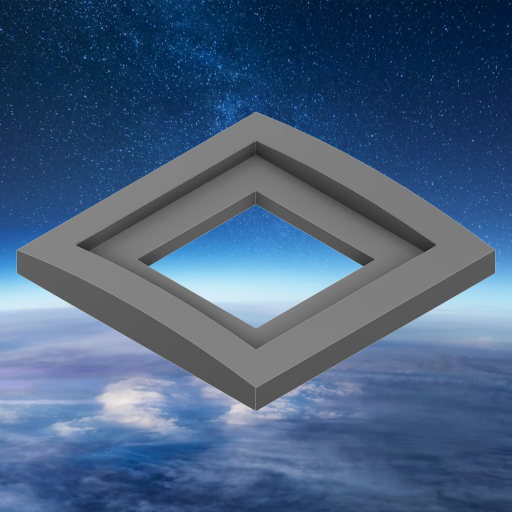
# Autodesk Inventor part: cooler_plate_socket
Saved by Autodesk Inventor 2023 (Build 270158000, 158)
## iProperties
Created: 2023-09-08
Part Number: cooler_plate_socket
Material: Acetal Resin, Black
Document SubType Name: Modeling
Designer: 310611102
Density: 1.425 g/cm^3
Appearance: Smooth - Black
Mass: 5.54751 g
Surface Area: 34.9135 cm^2
Volume: 3.89299 cm^3
Author: 310611102
Autodesk Inventor part; units mm, degrees
ref_plane "YZ Plane" through (0, 0, 0) normal (1, 0, 0) x (0, 1, 0)
ref_plane "XZ Plane" through (0, 0, 0) normal (0, 1, 0) x (-1, 0, 0)
ref_plane "XY Plane" through (0, 0, 0) normal (0, 0, 1) x (1, 0, 0)
sketch "Sketch1" plane through (0, 0, 0) normal (0, 0, 1) x (1, 0, 0)
  arc A0 (20, 123.3896) -> (-20, 123.3896) centre (0, 0) ccw
  line L0 (20, 120) -> (-20, 120)
  line L1 (-20, 120) -> (-20, 123.3896)
  line L2 (20, 120) -> (20, 123.3896)
  line L3 (0, 0) -> (0, 32.1156) construction
  point P0 (0, 125)
  dimension "d0" = 250
  dimension "d1" = 40
  dimension "d2" = 5
  constraints: 8 end point, 3 point on circle, 1 centre point, 1 coincident, 1 horizontal, 1 parallel, 1 perpendicular, 1 vertical, 1 other
  measures "d0" diameter of A0
  measures "d1" distance of L0.start L0.end
  measures "d2" distance from line of point (0, 125) L0
extrude "Extrusion1" add sketch "Sketch1" along normal blind 40
sketch "Sketch2" plane through (-20, 120, 0) normal (0, -1, 0) x (1, 0, 0)
  line L0 (4.85, 4.85) -> (35.15, 4.85)
  line L1 (35.15, 4.85) -> (35.15, 35.15)
  line L2 (35.15, 35.15) -> (4.85, 35.15)
  line L3 (4.85, 35.15) -> (4.85, 4.85)
  line L4 (4.85, 4.85) -> (35.15, 35.15) construction
  line L5 (35.15, 4.85) -> (4.85, 35.15) construction
  line L6 (40, 0) -> (40, 40) projected
  line L7 (40, 0) -> (0, 0) projected
  point P0 (20, 0)
  point P1 (20, 20)
  point P2 (40, 20)
  point P3 (20, 0)
  dimension "d6" = 30.3
  dimension "d7" = 30.3
  constraints: 12 end point, 4 midpoint, 2 parallel, 1 horizontal, 1 horizontal alignment, 1 perpendicular, 1 vertical alignment
  measures "d6" distance of L0.end L1.end
  measures "d7" distance of L0.start L0.end
extrude "Extrusion2" cut sketch "Sketch2" against normal blind 30
sketch "Sketch3" plane through (-20, 120, 0) normal (0, -1, 0) x (1, 0, 0)
  line L0 (35.15, 35.15) -> (35.15, 4.85) projected
  line L1 (4.85, 35.15) -> (35.15, 35.15)
  line L2 (35.15, 35.15) -> (35.15, 4.85)
  line L3 (35.15, 4.85) -> (4.85, 4.85)
  line L4 (4.85, 4.85) -> (4.85, 35.15)
  line L5 (4.85, 35.15) -> (35.15, 4.85) construction
  line L6 (35.15, 35.15) -> (4.85, 4.85) construction
  line L7 (10, 10) -> (30, 10)
  line L8 (30, 10) -> (30, 30)
  line L9 (30, 30) -> (10, 30)
  line L10 (10, 30) -> (10, 10)
  line L11 (10, 10) -> (30, 30) construction
  line L12 (30, 10) -> (10, 30) construction
  point P0 (20, 0)
  point P1 (20, 20)
  dimension "d10" = 20
  constraints: 24 end point, 4 midpoint, 4 parallel, 2 horizontal, 2 perpendicular, 1 coincident, 1 point on line
  measures "d10" distance of L8.end L9.end
extrude "Extrusion3" add sketch "Sketch3" against normal blind 2
body "Solid1"
